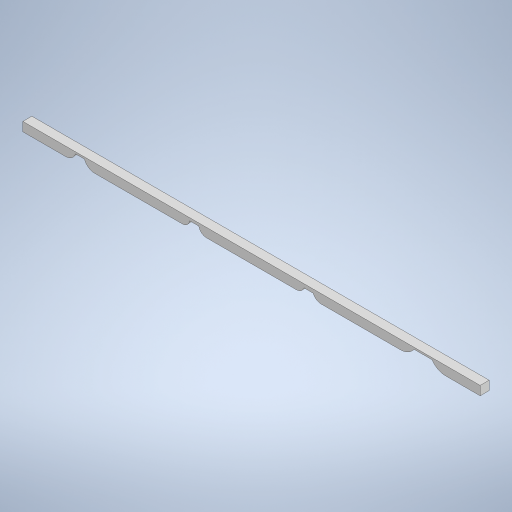
# Autodesk Inventor part: Hingetest
Saved by Autodesk Inventor 2023.1 (Build 271208000, 208)
## iProperties
Created: 2022-09-22
Part Number: Hingetest
Material: Generic
Document SubType Name: Modeling
Designer: Grimm
Density: 1 g/cm^3
Appearance: Default
Author: Grimm
Autodesk Inventor part; units mm, degrees
ref_plane "YZ Plane" through (0, 0, 0) normal (1, 0, 0) x (0, 1, 0)
ref_plane "XZ Plane" through (0, 0, 0) normal (0, 1, 0) x (-1, 0, 0)
ref_plane "XY Plane" through (0, 0, 0) normal (0, 0, 1) x (1, 0, 0)
sketch "Sketch1" plane through (0, 0, 0) normal (0, 0, 1) x (1, 0, 0)
  line L0 (-19.313, 5.3077) -> (234.687, 5.3077)
  line L1 (234.687, 5.3077) -> (234.687, 0.3077)
  line L2 (234.687, 0.3077) -> (-19.313, 0.3077)
  line L3 (-19.313, 0.3077) -> (-19.313, 5.3077)
  line L4 (44.187, 5.3077) -> (44.187, 0.3077) construction
  line L5 (171.187, 5.3077) -> (171.187, 0.3077) construction
  line L6 (107.687, 5.3077) -> (107.687, 0.3077) construction
  point P0 (0, 0)
  dimension "d0" = 254
  dimension "d1" = 5
  dimension "d2" = 63.5
  dimension "d3" = 63.5
  dimension "d4" = 63.5
  constraints: 14 end point, 4 perpendicular, 4 point on line, 2 midpoint, 2 parallel, 1 horizontal
  measures "d0" distance of L1.end L2.end
  measures "d1" distance of L0.end L1.end
  measures "d2" distance between parallel lines of L3 L4
  measures "d3" distance between parallel lines of L4 L6
  measures "d4" distance between parallel lines of L1 L5
extrude "Extrusion1" add sketch "Sketch1" along normal blind 5
sketch "Sketch2" plane through (0, 0, 0) normal (0, 0, -1) x (-1, 0, 0)
  line L0 (19.313, 0.3077) -> (-234.687, 0.3077) projected
  arc A0 (-20.4966, 0.3077) -> (-14.937, 4.3077) centre (-20.4966, 6.1713) ccw
  arc A1 (-9.937, 4.3077) -> (-4.3774, 0.3077) centre (-4.3774, 6.1713) ccw
  line L1 (-14.937, 4.3077) -> (-9.937, 4.3077)
  line L2 (19.313, 0.3077) -> (-234.687, 0.3077) projected
  line L3 (-234.687, 5.3077) -> (19.313, 5.3077) projected
  arc A2 (-82.7042, 0.3077) -> (-78.437, 3.8077) centre (-82.7042, 4.659) ccw
  arc A3 (-73.437, 3.8077) -> (-69.1698, 0.3077) centre (-69.1698, 4.659) ccw
  line L4 (-78.437, 3.8077) -> (-73.437, 3.8077)
  arc A4 (-146.3937, 0.3077) -> (-141.937, 3.3077) centre (-146.3937, 5.1181) ccw
  arc A5 (-136.937, 3.3077) -> (-132.4803, 0.3077) centre (-132.4803, 5.1181) ccw
  line L5 (-141.937, 3.3077) -> (-136.937, 3.3077)
  arc A6 (-215.504, 0.3077) -> (-207.937, 4.3077) centre (-215.504, 9.4651) ccw
  arc A7 (-197.937, 4.3077) -> (-190.37, 0.3077) centre (-190.37, 9.4651) ccw
  line L6 (-207.937, 4.3077) -> (-197.937, 4.3077)
  line L7 (19.313, 5.3077) -> (19.313, 0.3077) projected
  point P0 (0, 0)
  point P1 (19.313, 2.8077)
  point P2 (-12.437, 4.3077)
  point P3 (-75.937, 3.8077)
  point P4 (-139.437, 3.3077)
  point P5 (-202.937, 4.3077)
  point P6 (-82.7042, 0.3077)
  point P7 (-69.1698, 0.3077)
  point P8 (-146.3937, 0.3077)
  point P9 (-132.4803, 0.3077)
  point P10 (-215.504, 0.3077)
  point P11 (-190.37, 0.3077)
  dimension "d7" = 1
  dimension "d8" = 1.5
  dimension "d9" = 2
  dimension "d10" = 1
  dimension "d11" = 5
  dimension "d12" = 10
  dimension "d14" = 31.75
  dimension "d15" = 63.5
  dimension "d16" = 63.5
  dimension "d17" = 63.5
  constraints: 16 point on circle, 8 centre point, 8 end point, 5 midpoint, 5 tangent, 4 equal radius, 4 horizontal, 2 parallel, 2 point on line, 12 other
  measures "d7" distance between parallel lines of L3 L1
  measures "d8" distance between parallel lines of L3 L4
  measures "d9" distance between parallel lines of L3 L5
  measures "d10" distance between parallel lines of L3 L6
  measures "d11" distance of L1.start L1.end
  measures "d12" distance of L6.start L6.end
  measures "d14" distance from line of L7 point (-12.437, 4.308)
  measures "d15" horizontal distance of point (-12.437, 4.308) point (-75.937, 3.808)
  measures "d16" horizontal distance of point (-75.937, 3.808) point (-139.437, 3.308)
  measures "d17" horizontal distance of point (-139.437, 3.308) point (-202.937, 4.308)
extrude "Extrusion2" cut sketch "Sketch2" against normal through all
body "Solid1"
